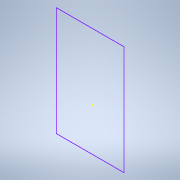
# Autodesk Inventor part: Corner
Saved by Autodesk Inventor 2022 (Build 260153000, 153)
## iProperties
Created: 2023-03-05
Part Number: Corner
Material: Generic
Document SubType Name: Modeling
Designer: Bunny
Density: 1 g/cm^3
Appearance: Default
Author: Bunny
Autodesk Inventor part; units mm, degrees
ref_plane "YZ Plane" through (0, 0, 0) normal (1, 0, 0) x (0, 1, 0)
ref_plane "XZ Plane" through (0, 0, 0) normal (0, 1, 0) x (-1, 0, 0)
ref_plane "XY Plane" through (0, 0, 0) normal (0, 0, 1) x (1, 0, 0)
sketch "Sketch1" plane through (0, 0, 0) normal (0, 0, 1) x (1, 0, 0)
  line L0 (-8.6606, 15.5596) -> (7.3394, 15.5596)
  line L1 (7.3394, 15.5596) -> (7.3394, -64.4404)
  line L2 (7.3394, -64.4404) -> (-8.6606, -64.4404)
  line L3 (-8.6606, -64.4404) -> (-8.6606, 15.5596)
  point P0 (0, 0)
  dimension "d2" = 16
  dimension "d3" = 80
  constraints: 8 end point, 2 parallel, 1 horizontal, 1 perpendicular
  measures "d2" distance of L0.start L0.end
  measures "d3" distance of L0.end L1.end
extrude "Extrusion1" add sketch "Sketch1" along normal blind 16
sketch "Sketch2" plane through (-8.6606, 15.5596, 0) normal (0, 1, 0) x (1, 0, 0)
  line L0 (16, 0) -> (16, -16) projected
  line L1 (16, -11) -> (11, -11)
  line L2 (11, -11) -> (11, -5)
  line L3 (11, -5) -> (16, -5)
  line L4 (16, -5) -> (16, -11)
  line L5 (16, 0) -> (0, 0) projected
  line L6 (5, 0) -> (11, 0)
  line L7 (11, 0) -> (11, -5)
  line L8 (11, -5) -> (5, -5)
  line L9 (5, -5) -> (5, 0)
  line L10 (16, -16) -> (0, -16) projected
  line L11 (0, 0) -> (0, -16) projected
  point P0 (8.6606, 0)
  point P1 (5, -16)
  point P2 (0, -11)
  dimension "d5" = 5
  dimension "d6" = 5
  dimension "d7" = 5
  dimension "d8" = 5
  dimension "d9" = 5
  dimension "d10" = 5
  constraints: 16 end point, 4 parallel, 2 horizontal, 2 perpendicular, 2 point on line
  measures "d5" distance between parallel lines of L10 L1
  measures "d6" distance between parallel lines of L5 L3
  measures "d7" distance of L2.end L3.end
  measures "d8" distance between parallel lines of L0 L7
  measures "d9" distance between parallel lines of L11 L9
  measures "d10" distance of L8.end L6.start
extrude "Extrusion2" cut sketch "Sketch2" against normal blind 80 contours L0 L3 L7 L5 | L0 L1 L2 L3 | L7 L8 L9 L5
sketch "Sketch4" plane through (-8.6606, 15.5596, 16) normal (0, 1, 0) x (1, 0, 0)
  line L0 (6.9788, 8.1833) -> (8.6242, 5.3333)
  line L1 (8.6242, 5.3333) -> (6.9788, 2.4833)
  line L2 (6.9788, 2.4833) -> (3.6879, 2.4833)
  line L3 (3.6879, 2.4833) -> (2.0424, 5.3333)
  line L4 (2.0424, 5.3333) -> (3.6879, 8.1833)
  line L5 (3.6879, 8.1833) -> (6.9788, 8.1833)
  line L6 (16, 0) -> (0, 0) projected
  line L7 (0, 16) -> (0, 0) projected
  point P0 (8.6606, 16)
  point P1 (5.3333, 5.3333)
  dimension "d13" = 5.3333
  dimension "d14" = 5.3333
  dimension "d15" = 5.7
  constraints: 12 end point, 1 parallel, 13 other
  measures "d13" distance from line of L7 point (5.333, 5.333)
  measures "d14" distance from line of L6 point (5.333, 5.333)
  measures "d15" distance between parallel lines of L2 L5
extrude "Extrusion3" cut sketch "Sketch4" against normal blind 2.7
sketch "Sketch5" plane through (-8.6606, -64.4404, 16) normal (0, -1, 0) x (1, 0, 0)
  line L0 (3.6879, -2.4833) -> (2.0424, -5.3333) projected
  line L1 (3.6879, -2.4833) -> (6.9788, -2.4833)
  line L2 (6.9788, -2.4833) -> (8.6242, -5.3333)
  line L3 (8.6242, -5.3333) -> (6.9788, -8.1833)
  line L4 (6.9788, -8.1833) -> (3.6879, -8.1833)
  line L5 (3.6879, -8.1833) -> (2.0424, -5.3333)
  line L6 (2.0424, -5.3333) -> (3.6879, -2.4833)
  line L7 (0, 0) -> (16, 0) projected
  line L8 (0, -16) -> (0, 0) projected
  point P0 (8.6606, -16)
  point P1 (5.3333, -5.3333)
  dimension "d18" = 5.3333
  dimension "d19" = 5.3333
  constraints: 12 end point, 1 parallel, 13 other
  measures "d18" distance from line of L7 point (5.333, -5.333)
  measures "d19" distance from line of L8 point (5.333, -5.333)
extrude "Extrusion4" cut sketch "Sketch5" against normal blind 2.7
fillet "Fillet2" radius 5 1 edges at (-8.6606, -24.4404, 16)
equation "\"d2\" = SheetThickness + 2 * CornerOffset"
equation "\"d3\" = BoxHeight"
equation "\"d0\" = SheetThickness + 2 * CornerOffset"
equation "\"d5\" = CornerOffset"
equation "\"d6\" = CornerOffset"
equation "\"d7\" = CornerOffset"
equation "\"d8\" = CornerOffset"
equation "\"d9\" = CornerOffset"
equation "\"d10\" = CornerOffset"
equation "\"d11\" = BoxHeight"
equation "\"d13\" = 0.666667 * CornerOffset + 0.333333 * SheetThickness"
equation "\"d14\" = 0.666667 * CornerOffset + 0.333333 * SheetThickness"
equation "\"d15\" = NutS"
equation "\"d16\" = NutM"
equation "\"d18\" = 0.666667 * CornerOffset + 0.333333 * SheetThickness"
equation "\"d20\" = NutM"
equation "\"BoxHeight\" = 80"
equation "\"SheetThickness\" = 6"
equation "\"CornerOffset\" = 5"
equation "\"NutM\" = 2.7"
equation "\"NutS\" = 5.7"
body "Solid1"
